Autodesk Fusion 360 part; units mm, degrees
(part 8 of 9)
  line L168 (107.3, 3.525) -> (107.3, 15.525)
  arc A160 (179.7375, 54.625) -> (178.7375, 53.625) centre (179.7375, 53.625) ccw
  line L169 (179.7375, 54.625) -> (191.7375, 54.625)
  arc A161 (192.7375, 53.625) -> (191.7375, 54.625) centre (191.7375, 53.625) ccw
  line L170 (192.7375, 53.625) -> (192.7375, 41.625)
  arc A162 (191.7375, 40.625) -> (192.7375, 41.625) centre (191.7375, 41.625) ccw
  line L171 (191.7375, 40.625) -> (179.7375, 40.625)
  arc A163 (178.7375, 41.625) -> (179.7375, 40.625) centre (179.7375, 41.625) ccw
  line L172 (178.7375, 41.625) -> (178.7375, 53.625)
  arc A164 (217.8375, 54.625) -> (216.8375, 53.625) centre (217.8375, 53.625) ccw
  line L173 (217.8375, 54.625) -> (229.8375, 54.625)
  arc A165 (230.8375, 53.625) -> (229.8375, 54.625) centre (229.8375, 53.625) ccw
  line L174 (230.8375, 53.625) -> (230.8375, 41.625)
  arc A166 (229.8375, 40.625) -> (230.8375, 41.625) centre (229.8375, 41.625) ccw
  line L175 (229.8375, 40.625) -> (217.8375, 40.625)
  arc A167 (216.8375, 41.625) -> (217.8375, 40.625) centre (217.8375, 41.625) ccw
  line L176 (216.8375, 41.625) -> (216.8375, 53.625)
  line L177 (229.1688, 22.575) -> (229.1688, 36.575)
  arc A168 (230.1688, 37.575) -> (229.1688, 36.575) centre (230.1688, 36.575) ccw
  line L178 (230.1688, 37.575) -> (236.1688, 37.575)
  arc A169 (237.1688, 36.575) -> (236.1688, 37.575) centre (236.1687, 36.575) ccw
  line L179 (237.1688, 36.575) -> (237.1688, 35.575)
  line L180 (237.1688, 35.575) -> (242.7688, 35.575)
  arc A170 (243.7688, 36.575) -> (242.7688, 35.575) centre (243.7688, 35.575) ccw
  line L181 (243.7688, 36.575) -> (246.7688, 36.575)
  arc A171 (247.7688, 35.575) -> (246.7688, 36.575) centre (246.7688, 35.575) ccw
  line L182 (247.7688, 35.575) -> (253.3688, 35.575)
  line L183 (253.3688, 35.575) -> (253.3688, 36.575)
  arc A172 (254.3688, 37.575) -> (253.3688, 36.575) centre (254.3688, 36.575) ccw
  line L184 (254.3688, 37.575) -> (260.3688, 37.575)
  arc A173 (261.3688, 36.575) -> (260.3688, 37.575) centre (260.3688, 36.575) ccw
  line L185 (261.3688, 36.575) -> (261.3688, 22.575)
  arc A174 (261.3687, 22.5664) -> (261.3688, 22.575) centre (260.3688, 22.575) ccw
  line L186 (261.3687, 22.5664) -> (261.3688, 22.5664)
  arc A175 (262.3688, 21.5664) -> (261.3688, 22.5664) centre (261.3688, 21.5664) ccw
  line L187 (262.3688, 21.5664) -> (262.3688, 16.525)
  line L188 (262.3688, 16.525) -> (263.175, 16.525)
  arc A176 (264.175, 15.525) -> (263.175, 16.525) centre (263.175, 15.525) ccw
  line L189 (264.175, 15.525) -> (264.175, 3.525)
  arc A177 (263.175, 2.525) -> (264.175, 3.525) centre (263.175, 3.525) ccw
  line L190 (263.175, 2.525) -> (251.175, 2.525)
  arc A178 (250.175, 3.525) -> (251.175, 2.525) centre (251.175, 3.525) ccw
  line L191 (250.175, 3.525) -> (250.175, 15.525)
  arc A179 (250.175, 15.525) -> (249.175, 16.525) centre (249.175, 15.525) ccw
  line L192 (249.175, 16.525) -> (241.3625, 16.525)
  arc A180 (241.3625, 16.525) -> (240.3625, 15.525) centre (241.3625, 15.525) ccw
  line L193 (240.3625, 15.525) -> (240.3625, 3.525)
  arc A181 (239.3625, 2.525) -> (240.3625, 3.525) centre (239.3625, 3.525) ccw
  line L194 (239.3625, 2.525) -> (227.3625, 2.525)
  arc A182 (226.3625, 3.525) -> (227.3625, 2.525) centre (227.3625, 3.525) ccw
  line L195 (226.3625, 3.525) -> (226.3625, 15.525)
  arc A183 (227.3625, 16.525) -> (226.3625, 15.525) centre (227.3625, 15.525) ccw
  line L196 (227.3625, 16.525) -> (228.1688, 16.525)
  line L197 (228.1688, 16.525) -> (228.1688, 21.5664)
  arc A184 (229.1688, 22.5664) -> (228.1688, 21.5664) centre (229.1688, 21.5664) ccw
  line L198 (229.1688, 22.5664) -> (229.1688, 22.5664)
  arc A185 (229.1688, 22.575) -> (229.1688, 22.5664) centre (230.1688, 22.575) ccw
  arc A186 (132.1125, 35.575) -> (131.1125, 34.575) centre (132.1125, 34.575) ccw
  line L199 (132.1125, 35.575) -> (144.1125, 35.575)
  arc A187 (145.1125, 34.575) -> (144.1125, 35.575) centre (144.1125, 34.575) ccw
  line L200 (145.1125, 34.575) -> (145.1125, 22.575)
  arc A188 (144.1125, 21.575) -> (145.1125, 22.575) centre (144.1125, 22.575) ccw
  line L201 (144.1125, 21.575) -> (132.1125, 21.575)
  arc A189 (131.1125, 22.575) -> (132.1125, 21.575) centre (132.1125, 22.575) ccw
  line L202 (131.1125, 22.575) -> (131.1125, 34.575)
  arc A190 (94.0125, 35.575) -> (93.0125, 34.575) centre (94.0125, 34.575) ccw
  line L203 (94.0125, 35.575) -> (106.0125, 35.575)
  arc A191 (107.0125, 34.575) -> (106.0125, 35.575) centre (106.0125, 34.575) ccw
  line L204 (107.0125, 34.575) -> (107.0125, 22.575)
  arc A192 (106.0125, 21.575) -> (107.0125, 22.575) centre (106.0125, 22.575) ccw
  line L205 (106.0125, 21.575) -> (94.0125, 21.575)
  arc A193 (93.0125, 22.575) -> (94.0125, 21.575) centre (94.0125, 22.575) ccw
  line L206 (93.0125, 22.575) -> (93.0125, 34.575)
  circle A194 centre (128.588, 37.025) radius 2
  circle A195 centre (220.025, 66.675) radius 2
  circle A196 centre (47.625, 9.525) radius 2
  circle A197 centre (245.269, 9.525) radius 2
  circle A198 centre (32.525, 66.675) radius 2
  line L207 (18.9313, 59.675) -> (23.9313, 59.675)
  line L208 (23.9313, 59.675) -> (23.9313, 58.675)
  line L209 (23.9313, 58.675) -> (18.9313, 58.675)
  line L210 (18.9313, 58.675) -> (18.9313, 59.675)
  line L211 (18.9313, 73.675) -> (23.9313, 73.675)
  line L212 (23.9313, 73.675) -> (23.9313, 74.675)
  line L213 (23.9313, 74.675) -> (18.9313, 74.675)
  line L214 (18.9313, 74.675) -> (18.9313, 73.675)
  line L215 (45.125, 59.675) -> (50.125, 59.675)
  line L216 (50.125, 59.675) -> (50.125, 58.675)
  line L217 (50.125, 58.675) -> (45.125, 58.675)
  line L218 (45.125, 58.675) -> (45.125, 59.675)
  line L219 (45.125, 73.675) -> (50.125, 73.675)
  line L220 (50.125, 73.675) -> (50.125, 74.675)
  line L221 (50.125, 74.675) -> (45.125, 74.675)
  line L222 (45.125, 74.675) -> (45.125, 73.675)
  line L223 (71.3188, 73.675) -> (76.3188, 73.675)
  line L224 (76.3188, 73.675) -> (76.3188, 74.675)
  line L225 (76.3188, 74.675) -> (71.3188, 74.675)
  line L226 (71.3188, 74.675) -> (71.3188, 73.675)
  line L227 (71.3188, 59.675) -> (76.3188, 59.675)
  line L228 (76.3188, 59.675) -> (76.3188, 58.675)
  line L229 (76.3188, 58.675) -> (71.3188, 58.675)
  line L230 (71.3188, 58.675) -> (71.3188, 59.675)
  line L231 (176.0937, 73.675) -> (181.0937, 73.675)
  line L232 (181.0937, 73.675) -> (181.0937, 74.675)
  line L233 (181.0937, 74.675) -> (176.0937, 74.675)
  line L234 (176.0937, 74.675) -> (176.0937, 73.675)
  line L235 (176.0938, 59.675) -> (181.0938, 59.675)
  line L236 (181.0938, 59.675) -> (181.0938, 58.675)
  line L237 (181.0938, 58.675) -> (176.0938, 58.675)
  line L238 (176.0938, 58.675) -> (176.0938, 59.675)
  line L239 (202.2875, 59.675) -> (207.2875, 59.675)
  line L240 (207.2875, 59.675) -> (207.2875, 58.675)
  line L241 (207.2875, 58.675) -> (202.2875, 58.675)
  line L242 (202.2875, 58.675) -> (202.2875, 59.675)
  line L243 (202.2875, 73.675) -> (207.2875, 73.675)
  line L244 (207.2875, 73.675) -> (207.2875, 74.675)
  line L245 (207.2875, 74.675) -> (202.2875, 74.675)
  line L246 (202.2875, 74.675) -> (202.2875, 73.675)
  line L247 (228.4813, 73.675) -> (233.4813, 73.675)
  line L248 (233.4813, 73.675) -> (233.4813, 74.675)
  line L249 (233.4813, 74.675) -> (228.4813, 74.675)
  line L250 (228.4813, 74.675) -> (228.4813, 73.675)
  line L251 (228.4812, 59.675) -> (233.4812, 59.675)
  line L252 (233.4812, 59.675) -> (233.4812, 58.675)
  line L253 (233.4812, 58.675) -> (228.4812, 58.675)
  line L254 (228.4812, 58.675) -> (228.4812, 59.675)
  line L255 (247.5312, 54.625) -> (252.5312, 54.625)
  line L256 (252.5312, 54.625) -> (252.5312, 55.625)
  line L257 (252.5312, 55.625) -> (247.5312, 55.625)
  line L258 (247.5312, 55.625) -> (247.5312, 54.625)
  line L259 (252.5312, 40.625) -> (247.5312, 40.625)
  line L260 (247.5312, 40.625) -> (247.5312, 39.625)
  line L261 (247.5312, 39.625) -> (252.5312, 39.625)
  line L262 (252.5312, 39.625) -> (252.5312, 40.625)
  line L263 (221.3375, 40.625) -> (226.3375, 40.625)
  line L264 (226.3375, 40.625) -> (226.3375, 39.625)
  line L265 (226.3375, 39.625) -> (221.3375, 39.625)
  line L266 (221.3375, 39.625) -> (221.3375, 40.625)
  line L267 (221.3375, 54.625) -> (226.3375, 54.625)
  line L268 (226.3375, 54.625) -> (226.3375, 55.625)
  line L269 (226.3375, 55.625) -> (221.3375, 55.625)
  line L270 (221.3375, 55.625) -> (221.3375, 54.625)
  line L271 (202.2875, 54.625) -> (207.2875, 54.625)
  line L272 (207.2875, 54.625) -> (207.2875, 55.625)
  line L273 (207.2875, 55.625) -> (202.2875, 55.625)
  line L274 (202.2875, 55.625) -> (202.2875, 54.625)
  line L275 (202.2875, 40.625) -> (207.2875, 40.625)
  line L276 (207.2875, 40.625) -> (207.2875, 39.625)
  line L277 (207.2875, 39.625) -> (202.2875, 39.625)
  line L278 (202.2875, 39.625) -> (202.2875, 40.625)
  line L279 (183.2375, 54.625) -> (188.2375, 54.625)
  line L280 (188.2375, 54.625) -> (188.2375, 55.625)
  line L281 (188.2375, 55.625) -> (183.2375, 55.625)
  line L282 (183.2375, 55.625) -> (183.2375, 54.625)
  line L283 (183.2375, 40.625) -> (188.2375, 40.625)
  line L284 (188.2375, 40.625) -> (188.2375, 39.625)
  line L285 (188.2375, 39.625) -> (183.2375, 39.625)
  line L286 (183.2375, 39.625) -> (183.2375, 40.625)
  line L287 (164.1875, 40.625) -> (169.1875, 40.625)
  line L288 (169.1875, 40.625) -> (169.1875, 39.625)
  line L289 (169.1875, 39.625) -> (164.1875, 39.625)
  line L290 (164.1875, 39.625) -> (164.1875, 40.625)
  line L291 (254.675, 2.525) -> (259.675, 2.525)
  line L292 (259.675, 2.525) -> (259.675, 1.525)
  line L293 (259.675, 1.525) -> (254.675, 1.525)
  line L294 (254.675, 1.525) -> (254.675, 2.525)
  line L295 (230.8625, 2.525) -> (235.8625, 2.525)
  line L296 (235.8625, 2.525) -> (235.8625, 1.525)
  line L297 (235.8625, 1.525) -> (230.8625, 1.525)
  line L298 (230.8625, 1.525) -> (230.8625, 2.525)
  line L299 (207.05, 2.525) -> (212.05, 2.525)
  line L300 (212.05, 2.525) -> (212.05, 1.525)
  line L301 (212.05, 1.525) -> (207.05, 1.525)
  line L302 (207.05, 1.525) -> (207.05, 2.525)
  line L303 (207.05, 16.525) -> (212.05, 16.525)
  line L304 (212.05, 16.525) -> (212.05, 17.525)
  line L305 (212.05, 17.525) -> (207.05, 17.525)
  line L306 (207.05, 17.525) -> (207.05, 16.525)
  line L307 (211.8125, 35.575) -> (216.8125, 35.575)
  line L308 (216.8125, 35.575) -> (216.8125, 36.575)
  line L309 (216.8125, 36.575) -> (211.8125, 36.575)
  line L310 (211.8125, 36.575) -> (211.8125, 35.575)
  line L311 (211.8125, 21.575) -> (216.8125, 21.575)
  line L312 (216.8125, 21.575) -> (216.8125, 20.575)
  line L313 (216.8125, 20.575) -> (211.8125, 20.575)
  line L314 (211.8125, 20.575) -> (211.8125, 21.575)
  line L315 (192.7625, 35.575) -> (197.7625, 35.575)
  line L316 (197.7625, 35.575) -> (197.7625, 36.575)
  line L317 (197.7625, 36.575) -> (192.7625, 36.575)
  line L318 (192.7625, 36.575) -> (192.7625, 35.575)
  line L319 (192.7625, 21.575) -> (197.7625, 21.575)
  line L320 (197.7625, 21.575) -> (197.7625, 20.575)
  line L321 (197.7625, 20.575) -> (192.7625, 20.575)
  line L322 (192.7625, 20.575) -> (192.7625, 21.575)
  line L323 (188, 16.525) -> (193, 16.525)
  line L324 (193, 16.525) -> (193, 17.525)
  line L325 (193, 17.525) -> (188, 17.525)
  line L326 (188, 17.525) -> (188, 16.525)
  line L327 (188, 2.525) -> (193, 2.525)
  line L328 (193, 2.525) -> (193, 1.525)
  line L329 (193, 1.525) -> (188, 1.525)
  line L330 (188, 1.525) -> (188, 2.525)
  line L331 (173.7125, 35.575) -> (178.7125, 35.575)
  line L332 (178.7125, 35.575) -> (178.7125, 36.575)
  line L333 (178.7125, 36.575) -> (173.7125, 36.575)
  line L334 (173.7125, 36.575) -> (173.7125, 35.575)
  line L335 (173.7125, 21.575) -> (178.7125, 21.575)
  line L336 (178.7125, 21.575) -> (178.7125, 20.575)
  line L337 (178.7125, 20.575) -> (173.7125, 20.575)
  line L338 (173.7125, 20.575) -> (173.7125, 21.575)
  line L339 (168.95, 16.525) -> (173.95, 16.525)
  line L340 (173.95, 16.525) -> (173.95, 17.525)
  line L341 (173.95, 17.525) -> (168.95, 17.525)
  line L342 (168.95, 17.525) -> (168.95, 16.525)
  line L343 (168.95, 2.525) -> (173.95, 2.525)
  line L344 (173.95, 2.525) -> (173.95, 1.525)
  line L345 (173.95, 1.525) -> (168.95, 1.525)
  line L346 (168.95, 1.525) -> (168.95, 2.525)
  line L347 (149.9, 16.525) -> (154.9, 16.525)
  line L348 (154.9, 16.525) -> (154.9, 17.525)
  line L349 (154.9, 17.525) -> (149.9, 17.525)
  line L350 (149.9, 17.525) -> (149.9, 16.525)
  line L351 (149.9, 2.525) -> (154.9, 2.525)
  line L352 (154.9, 2.525) -> (154.9, 1.525)
  line L353 (154.9, 1.525) -> (149.9, 1.525)
  line L354 (149.9, 1.525) -> (149.9, 2.525)
  line L355 (154.6625, 35.575) -> (159.6625, 35.575)
  line L356 (159.6625, 35.575) -> (159.6625, 36.575)
  line L357 (159.6625, 36.575) -> (154.6625, 36.575)
  line L358 (154.6625, 36.575) -> (154.6625, 35.575)
  line L359 (154.6625, 21.575) -> (159.6625, 21.575)
  line L360 (159.6625, 21.575) -> (159.6625, 20.575)
  line L361 (159.6625, 20.575) -> (154.6625, 20.575)
  line L362 (154.6625, 20.575) -> (154.6625, 21.575)
  line L363 (145.1375, 40.625) -> (150.1375, 40.625)
  line L364 (150.1375, 40.625) -> (150.1375, 39.625)
  line L365 (150.1375, 39.625) -> (145.1375, 39.625)
  line L366 (145.1375, 39.625) -> (145.1375, 40.625)
  line L367 (135.6125, 35.575) -> (140.6125, 35.575)
  line L368 (140.6125, 35.575) -> (140.6125, 36.575)
  line L369 (140.6125, 36.575) -> (135.6125, 36.575)
  line L370 (135.6125, 36.575) -> (135.6125, 35.575)
  line L371 (126.0875, 40.625) -> (131.0875, 40.625)
  line L372 (131.0875, 40.625) -> (131.0875, 39.625)
  line L373 (131.0875, 39.625) -> (126.0875, 39.625)
  line L374 (126.0875, 39.625) -> (126.0875, 40.625)
  line L375 (135.6125, 21.575) -> (140.6125, 21.575)
  line L376 (140.6125, 21.575) -> (140.6125, 20.575)
  line L377 (140.6125, 20.575) -> (135.6125, 20.575)
  line L378 (135.6125, 20.575) -> (135.6125, 21.575)
  line L379 (130.85, 16.525) -> (135.85, 16.525)
  line L380 (135.85, 16.525) -> (135.85, 17.525)
  line L381 (135.85, 17.525) -> (130.85, 17.525)
  line L382 (130.85, 17.525) -> (130.85, 16.525)
  line L383 (130.85, 2.525) -> (135.85, 2.525)
  line L384 (135.85, 2.525) -> (135.85, 1.525)
  line L385 (135.85, 1.525) -> (130.85, 1.525)
  line L386 (130.85, 1.525) -> (130.85, 2.525)
  line L387 (107.0375, 40.625) -> (112.0375, 40.625)
  line L388 (112.0375, 40.625) -> (112.0375, 39.625)
  line L389 (112.0375, 39.625) -> (107.0375, 39.625)
  line L390 (107.0375, 39.625) -> (107.0375, 40.625)
  line L391 (87.9875, 40.625) -> (92.9875, 40.625)
  line L392 (92.9875, 40.625) -> (92.9875, 39.625)
  line L393 (92.9875, 39.625) -> (87.9875, 39.625)
  line L394 (87.9875, 39.625) -> (87.9875, 40.625)
  line L395 (97.5125, 35.575) -> (102.5125, 35.575)
  line L396 (102.5125, 35.575) -> (102.5125, 36.575)
  line L397 (102.5125, 36.575) -> (97.5125, 36.575)
  line L398 (97.5125, 36.575) -> (97.5125, 35.575)
  line L399 (116.5625, 35.575) -> (121.5625, 35.575)
  line L400 (121.5625, 35.575) -> (121.5625, 36.575)
  line L401 (121.5625, 36.575) -> (116.5625, 36.575)
  line L402 (116.5625, 36.575) -> (116.5625, 35.575)
  line L403 (116.5625, 21.575) -> (121.5625, 21.575)
  line L404 (121.5625, 21.575) -> (121.5625, 20.575)
  line L405 (121.5625, 20.575) -> (116.5625, 20.575)
  line L406 (116.5625, 20.575) -> (116.5625, 21.575)
  line L407 (97.5125, 21.575) -> (102.5125, 21.575)
  line L408 (102.5125, 21.575) -> (102.5125, 20.575)
  line L409 (102.5125, 20.575) -> (97.5125, 20.575)
  line L410 (97.5125, 20.575) -> (97.5125, 21.575)
  line L411 (92.75, 16.525) -> (97.75, 16.525)
  line L412 (97.75, 16.525) -> (97.75, 17.525)
  line L413 (97.75, 17.525) -> (92.75, 17.525)
  line L414 (92.75, 17.525) -> (92.75, 16.525)
  line L415 (92.75, 2.525) -> (97.75, 2.525)
  line L416 (97.75, 2.525) -> (97.75, 1.525)
  line L417 (97.75, 1.525) -> (92.75, 1.525)
  line L418 (92.75, 1.525) -> (92.75, 2.525)
  line L419 (111.8, 16.525) -> (116.8, 16.525)
  line L420 (116.8, 16.525) -> (116.8, 17.525)
  line L421 (116.8, 17.525) -> (111.8, 17.525)
  line L422 (111.8, 17.525) -> (111.8, 16.525)
  line L423 (111.8, 2.525) -> (116.8, 2.525)
  line L424 (116.8, 2.525) -> (116.8, 1.525)
  line L425 (116.8, 1.525) -> (111.8, 1.525)
  line L426 (111.8, 1.525) -> (111.8, 2.525)
  line L427 (68.9375, 54.625) -> (73.9375, 54.625)
  line L428 (73.9375, 54.625) -> (73.9375, 55.625)
  line L429 (73.9375, 55.625) -> (68.9375, 55.625)
  line L430 (68.9375, 55.625) -> (68.9375, 54.625)
  line L431 (49.8875, 54.625) -> (54.8875, 54.625)
  line L432 (54.8875, 54.625) -> (54.8875, 55.625)
  line L433 (54.8875, 55.625) -> (49.8875, 55.625)
  line L434 (49.8875, 55.625) -> (49.8875, 54.625)
  line L435 (49.8875, 40.625) -> (54.8875, 40.625)
  line L436 (54.8875, 40.625) -> (54.8875, 39.625)
  line L437 (54.8875, 39.625) -> (49.8875, 39.625)
  line L438 (49.8875, 39.625) -> (49.8875, 40.625)
  line L439 (68.9375, 40.625) -> (73.9375, 40.625)
  line L440 (73.9375, 40.625) -> (73.9375, 39.625)
  line L441 (73.9375, 39.625) -> (68.9375, 39.625)
  line L442 (68.9375, 39.625) -> (68.9375, 40.625)
  line L443 (14.1688, 21.575) -> (19.1688, 21.575)
  line L444 (19.1688, 21.575) -> (19.1688, 20.575)
  line L445 (19.1688, 20.575) -> (14.1688, 20.575)
  line L446 (14.1688, 20.575) -> (14.1688, 21.575)
  line L447 (40.3625, 21.575) -> (45.3625, 21.575)
  line L448 (45.3625, 21.575) -> (45.3625, 20.575)
  line L449 (45.3625, 20.575) -> (40.3625, 20.575)
  line L450 (40.3625, 20.575) -> (40.3625, 21.575)
  line L451 (59.4125, 35.575) -> (64.4125, 35.575)
  line L452 (64.4125, 35.575) -> (64.4125, 36.575)
  line L453 (64.4125, 36.575) -> (59.4125, 36.575)
  line L454 (59.4125, 36.575) -> (59.4125, 35.575)
  line L455 (59.4125, 21.575) -> (64.4125, 21.575)
  line L456 (64.4125, 21.575) -> (64.4125, 20.575)
  line L457 (64.4125, 20.575) -> (59.4125, 20.575)
  line L458 (59.4125, 20.575) -> (59.4125, 21.575)
  line L459 (78.4625, 21.575) -> (83.4625, 21.575)
  line L460 (83.4625, 21.575) -> (83.4625, 20.575)
  line L461 (83.4625, 20.575) -> (78.4625, 20.575)
  line L462 (78.4625, 20.575) -> (78.4625, 21.575)
  line L463 (78.4625, 35.575) -> (83.4625, 35.575)
  line L464 (83.4625, 35.575) -> (83.4625, 36.575)
  line L465 (83.4625, 36.575) -> (78.4625, 36.575)
  line L466 (78.4625, 36.575) -> (78.4625, 35.575)
  line L467 (11.7875, 2.525) -> (16.7875, 2.525)
  line L468 (16.7875, 2.525) -> (16.7875, 1.525)
  line L469 (16.7875, 1.525) -> (11.7875, 1.525)
  line L470 (11.7875, 1.525) -> (11.7875, 2.525)
  line L471 (11.7875, 16.525) -> (16.7875, 16.525)
  line L472 (16.7875, 16.525) -> (16.7875, 17.525)
  line L473 (16.7875, 17.525) -> (11.7875, 17.525)
  line L474 (11.7875, 17.525) -> (11.7875, 16.525)
  line L475 (35.6, 16.525) -> (40.6, 16.525)
  line L476 (40.6, 16.525) -> (40.6, 17.525)
  line L477 (40.6, 17.525) -> (35.6, 17.525)
  line L478 (35.6, 17.525) -> (35.6, 16.525)
  line L479 (35.6, 2.525) -> (40.6, 2.525)
  line L480 (40.6, 2.525) -> (40.6, 1.525)
  line L481 (40.6, 1.525) -> (35.6, 1.525)
  line L482 (35.6, 1.525) -> (35.6, 2.525)
  line L483 (54.65, 2.525) -> (59.65, 2.525)
  line L484 (59.65, 2.525) -> (59.65, 1.525)
  line L485 (59.65, 1.525) -> (54.65, 1.525)
  line L486 (54.65, 1.525) -> (54.65, 2.525)
  line L487 (73.7, 2.525) -> (78.7, 2.525)
  line L488 (78.7, 2.525) -> (78.7, 1.525)
  line L489 (78.7, 1.525) -> (73.7, 1.525)
  line L490 (73.7, 1.525) -> (73.7, 2.525)
  line L491 (73.7, 16.525) -> (78.7, 16.525)
  line L492 (78.7, 16.525) -> (78.7, 17.525)
  line L493 (78.7, 17.525) -> (73.7, 17.525)
  line L494 (73.7, 17.525) -> (73.7, 16.525)
  line L495 (54.65, 16.525) -> (59.65, 16.525)
  line L496 (59.65, 16.525) -> (59.65, 17.525)
  line L497 (59.65, 17.525) -> (54.65, 17.525)
  line L498 (54.65, 17.525) -> (54.65, 16.525)
  dimension "d208" = 5
  dimension "d209" = 1
  dimension "d210" = 5
  dimension "d211" = 4.5
  dimension "d212" = 4.5
  dimension "d213" = 5
  dimension "d214" = 1
  dimension "d215" = 5
  dimension "d216" = 4.5
  dimension "d217" = 4.5
  dimension "d218" = 5
  dimension "d219" = 5
  dimension "d220" = 1
  dimension "d221" = 4.5
  dimension "d222" = 4.5
  dimension "d223" = 5
  dimension "d224" = 5
  dimension "d225" = 1
  dimension "d226" = 5
  dimension "d227" = 1
  dimension "d228" = 5
  dimension "d229" = 5
  dimension "d230" = 5
  dimension "d231" = 1
  dimension "d232" = 4.5
  dimension "d233" = 4.5
  dimension "d234" = 4.5
  dimension "d235" = 4.5
  dimension "d236" = 4.5
  dimension "d237" = 4.5
  dimension "d238" = 5
  dimension "d239" = 5
  dimension "d240" = 1
  dimension "d241" = 5
  dimension "d242" = 1
  dimension "d243" = 5
  dimension "d244" = 1
  dimension "d245" = 4.5
  dimension "d246" = 4.5
  dimension "d247" = 4.5
  dimension "d248" = 4.5
  dimension "d249" = 5
  dimension "d250" = 1
  dimension "d251" = 5
  dimension "d252" = 1
  dimension "d253" = 5
  dimension "d254" = 1
  dimension "d255" = 5
  dimension "d256" = 1
  dimension "d257" = 5
  dimension "d258" = 1
  dimension "d259" = 4.5
  dimension "d260" = 4.5
  dimension "d261" = 4.5
  dimension "d262" = 4.5
  dimension "d263" = 4.5
  dimension "d264" = 5
  dimension "d265" = 5
  dimension "d266" = 4.5
  dimension "d267" = 4.5
  dimension "d268" = 5
  dimension "d269" = 5
  dimension "d270" = 1
  dimension "d271" = 5
  dimension "d272" = 1
  dimension "d273" = 5
  dimension "d274" = 1
  dimension "d275" = 5
  dimension "d276" = 1
  dimension "d277" = 5
  dimension "d278" = 1
  dimension "d279" = 5
  dimension "d280" = 1
  dimension "d281" = 5
  dimension "d282" = 4.5
  dimension "d283" = 4.5
  dimension "d284" = 4.5
  dimension "d285" = 4.5
  dimension "d286" = 4.5
  dimension "d287" = 4.5
  dimension "d288" = 4.5
  dimension "d289" = 4.5
  dimension "d290" = 5
  dimension "d291" = 1
  dimension "d292" = 5
  dimension "d293" = 1
  dimension "d294" = 5
  dimension "d295" = 1
  dimension "d296" = 5
  dimension "d297" = 5
  dimension "d298" = 1
  dimension "d299" = 5
  dimension "d300" = 5
  dimension "d301" = 1
  dimension "d302" = 5
  dimension "d303" = 1
  dimension "d304" = 4.5
  dimension "d305" = 4.5
  dimension "d306" = 4.5
  dimension "d307" = 4.5
  dimension "d308" = 4.5
  dimension "d309" = 4.5
  dimension "d310" = 4.5
  dimension "d311" = 4.5
  dimension "d312" = 5
  dimension "d313" = 1
  dimension "d314" = 5
  dimension "d315" = 1
  dimension "d316" = 5
  dimension "d317" = 1
  dimension "d318" = 5
  dimension "d319" = 1
  dimension "d320" = 5
  dimension "d321" = 1
  dimension "d322" = 5
  dimension "d323" = 4.5
  dimension "d324" = 4.5
  dimension "d325" = 4.5
  dimension "d326" = 4.5
  dimension "d327" = 4.5
  dimension "d328" = 4.5
  dimension "d329" = 5
  dimension "d330" = 1
  dimension "d331" = 5
  dimension "d332" = 1
  dimension "d333" = 5
  dimension "d334" = 1
  dimension "d335" = 5
  dimension "d336" = 1
  dimension "d337" = 5
  dimension "d338" = 1
  dimension "d339" = 5
  dimension "d340" = 1
  dimension "d341" = 5
  dimension "d342" = 1
  dimension "d343" = 5
  dimension "d344" = 5
  dimension "d345" = 1
  dimension "d346" = 5
  dimension "d347" = 4.5
  dimension "d348" = 4.5
  dimension "d349" = 4.5
  dimension "d350" = 4.5
  dimension "d351" = 4.5
  dimension "d352" = 4.5
  dimension "d353" = 4.5
  dimension "d354" = 4.5
  dimension "d355" = 4.5
  dimension "d356" = 4.5
  dimension "d357" = 5
  dimension "d358" = 1
  dimension "d359" = 5
  dimension "d360" = 1
  dimension "d361" = 5
  dimension "d362" = 1
  dimension "d363" = 5
  dimension "d364" = 1
  dimension "d365" = 4.5
  dimension "d366" = 4.5
  dimension "d367" = 4.5
  dimension "d368" = 4.5
  dimension "d369" = 5
  dimension "d370" = 1
  dimension "d371" = 5
  dimension "d372" = 1
  dimension "d373" = 5
  dimension "d374" = 1
  dimension "d375" = 5
  dimension "d376" = 1
  dimension "d377" = 5
  dimension "d378" = 1
  dimension "d379" = 5
  dimension "d380" = 1
  dimension "d381" = 4.5
  dimension "d382" = 4.5
  dimension "d383" = 4.5
  dimension "d384" = 4.5
  dimension "d385" = 4.5
  dimension "d386" = 4.5
  dimension "d387" = 5
  dimension "d388" = 5
  dimension "d389" = 1
  dimension "d390" = 5
  dimension "d391" = 1
  dimension "d392" = 5
  dimension "d393" = 5
  dimension "d394" = 5
  dimension "d395" = 5
  dimension "d396" = 1
  dimension "d397" = 5
  dimension "d398" = 1
  dimension "d399" = 4.5
  dimension "d400" = 4.5
  dimension "d401" = 4.5
  dimension "d402" = 4.5
  dimension "d403" = 4.5
  dimension "d404" = 4.5
  dimension "d405" = 4.5
  dimension "d406" = 4.5
  constraint horizontal L207
  constraint vertical L208
  constraint horizontal L209
  constraint vertical L210
  constraint coincident L72 L207.start
  constraint horizontal L211
  constraint vertical L212
  constraint horizontal L213
  constraint vertical L214
  constraint coincident L70 L211.start
  constraint horizontal L215
  constraint vertical L216
  constraint horizontal L217
  constraint vertical L218
  constraint coincident L115 L215.start
  constraint horizontal L219
  constraint vertical L220
  constraint horizontal L221
  constraint vertical L222
  constraint coincident L113 L219.start
  constraint horizontal L223
  constraint vertical L224
  constraint horizontal L225
  constraint vertical L226
  constraint coincident L77 L223.start
  constraint horizontal L227
  constraint vertical L228
  constraint horizontal L229
  constraint vertical L230
  constraint coincident L79 L227.start
  constraint horizontal L231
  constraint vertical L232
  constraint horizontal L233
  constraint vertical L234
  constraint coincident L101 L231.start
  constraint horizontal L235
  constraint vertical L236
  constraint horizontal L237
  constraint vertical L238
  constraint coincident L103 L235.start
  constraint horizontal L239
  constraint vertical L240
  constraint horizontal L241
  constraint vertical L242
  constraint coincident L63 L239.start
  constraint horizontal L243
  constraint vertical L244
  constraint horizontal L245
  constraint vertical L246
  constraint coincident L61 L243.start
  constraint horizontal L247
  constraint vertical L248
  constraint horizontal L249
  constraint vertical L250
  constraint coincident L137 L247.start
  constraint horizontal L251
  constraint vertical L252
  constraint horizontal L253
  constraint vertical L254
  constraint coincident L139 L251.start
  constraint horizontal L255
  constraint vertical L256
  constraint horizontal L257
  constraint vertical L258
  constraint coincident L65 L255.start
  constraint horizontal L259
  constraint vertical L260
  constraint horizontal L261
  constraint vertical L262
  constraint coincident L67 L259.start
  constraint horizontal L263
  constraint vertical L264
  constraint horizontal L265
  constraint vertical L266
  constraint coincident L175 L263.start
  constraint horizontal L267
  constraint vertical L268
  constraint horizontal L269
  constraint vertical L270
  constraint coincident L173 L267.start
  constraint horizontal L271
  constraint vertical L272
  constraint horizontal L273
  constraint vertical L274
  constraint coincident L133 L271.start
  constraint horizontal L275
  constraint vertical L276
  constraint horizontal L277
  constraint vertical L278
  constraint coincident L135 L275.start
  constraint horizontal L279
  constraint vertical L280
  constraint horizontal L281
  constraint vertical L282
  constraint coincident L169 L279.start
  constraint horizontal L283
  constraint vertical L284
  constraint horizontal L285
  constraint vertical L286
  constraint coincident L171 L283.start
  constraint horizontal L287
  constraint vertical L288
  constraint horizontal L289
  constraint vertical L290
  constraint coincident L19 L287.start
  constraint horizontal L291
  constraint vertical L292
  constraint horizontal L293
  constraint vertical L294
  constraint coincident L190 L291.start
  constraint horizontal L295
  constraint vertical L296
  constraint horizontal L297
  constraint vertical L298
  constraint coincident L194 L295.start
  constraint horizontal L299
  constraint vertical L300
  constraint horizontal L301
  constraint vertical L302
  constraint coincident L163 L299.start
  constraint horizontal L303
  constraint vertical L304
  constraint horizontal L305
  constraint vertical L306
  constraint coincident L161 L303.start
  constraint horizontal L307
  constraint vertical L308
  constraint horizontal L309
  constraint vertical L310
  constraint coincident L121 L307.start
  constraint horizontal L311
  constraint vertical L312
  constraint horizontal L313
  constraint vertical L314
  constraint coincident L123 L311.start
  constraint horizontal L315
  constraint vertical L316
  constraint horizontal L317
  constraint vertical L318
  constraint coincident L157 L315.start
  constraint horizontal L319
  constraint vertical L320
  constraint horizontal L321
  constraint vertical L322
  constraint coincident L159 L319.start
  constraint horizontal L323
  constraint vertical L324
  constraint horizontal L325
  constraint vertical L326
  constraint coincident L81 L323.start
  constraint horizontal L327
  constraint vertical L328
  constraint horizontal L329
  constraint vertical L330
  constraint coincident L83 L327.start
  constraint horizontal L331
  constraint vertical L332
  constraint horizontal L333
  constraint vertical L334
  constraint coincident L141 L331.start
  constraint horizontal L335
  constraint vertical L336
  constraint horizontal L337
  constraint vertical L338
  constraint coincident L143 L335.start
  constraint horizontal L339
  constraint vertical L340
  constraint horizontal L341
  constraint vertical L342
  constraint coincident L73 L339.start
  constraint horizontal L343
  constraint vertical L344
  constraint horizontal L345
  constraint vertical L346
  constraint coincident L75 L343.start
  constraint horizontal L347
  constraint vertical L348
  constraint horizontal L349
  constraint vertical L350
  constraint coincident L153 L347.start
  constraint horizontal L351
  constraint vertical L352
  constraint horizontal L353
  constraint vertical L354
  constraint coincident L155 L351.start
  constraint horizontal L355
  constraint vertical L356
  constraint horizontal L357
  constraint vertical L358
  constraint coincident L105 L355.start
  constraint horizontal L359
  constraint vertical L360
  constraint horizontal L361
  constraint vertical L362
  constraint coincident L107 L359.start
  constraint horizontal L363
  constraint vertical L364
  constraint horizontal L365
  constraint vertical L366
  constraint coincident L23 L363.start
  constraint horizontal L367
  constraint vertical L368
  constraint horizontal L369
  constraint vertical L370
  constraint coincident L199 L367.start
  constraint horizontal L371
  constraint vertical L372
  constraint horizontal L373
  constraint vertical L374
  constraint coincident L27 L371.start
  constraint horizontal L375
  constraint vertical L376
  constraint horizontal L377
  constraint vertical L378
  constraint coincident L201 L375.start
  constraint horizontal L379
  constraint vertical L380
  constraint horizontal L381
  constraint vertical L382
  constraint coincident L145 L379.start
  constraint horizontal L383
  constraint vertical L384
  constraint horizontal L385
  constraint vertical L386
  constraint coincident L147 L383.start
  constraint horizontal L387
  constraint vertical L388
  constraint horizontal L389
  constraint vertical L390
  constraint coincident L31 L387.start
  constraint horizontal L391
  constraint vertical L392
  constraint horizontal L393
  constraint vertical L394
  constraint coincident L35 L391.start
  constraint horizontal L395
  constraint vertical L396
  constraint horizontal L397
  constraint vertical L398
  constraint coincident L203 L395.start
  constraint horizontal L399
  constraint vertical L400
  constraint horizontal L401
  constraint vertical L402
  constraint coincident L149 L399.start
  constraint horizontal L403
  constraint vertical L404
  constraint horizontal L405
  constraint vertical L406
  constraint coincident L151 L403.start
  constraint horizontal L407
  constraint vertical L408
  constraint horizontal L409
  constraint vertical L410
  constraint coincident L205 L407.start
  constraint horizontal L411
  constraint vertical L412
  constraint horizontal L413
  constraint vertical L414
  constraint coincident L109 L411.start
  constraint horizontal L415
  constraint vertical L416
  constraint horizontal L417
  constraint vertical L418
  constraint coincident L111 L415.start
  constraint horizontal L419
  constraint vertical L420
  constraint horizontal L421
  constraint vertical L422
  constraint coincident L165 L419.start
  constraint horizontal L423
  constraint vertical L424
  constraint horizontal L425
  constraint vertical L426
  constraint coincident L167 L423.start
  constraint horizontal L427
  constraint vertical L428
  constraint horizontal L429
  constraint vertical L430
  constraint coincident L57 L427.start
  constraint horizontal L431
  constraint vertical L432
  constraint horizontal L433
  constraint vertical L434
  constraint coincident L93 L431.start
  constraint horizontal L435
  constraint vertical L436
  constraint horizontal L437
  constraint vertical L438
  constraint coincident L95 L435.start
  constraint horizontal L439
  constraint vertical L440
  constraint horizontal L441
  constraint vertical L442
  constraint coincident L59 L439.start
  constraint horizontal L443
  constraint vertical L444
  constraint horizontal L445
  constraint vertical L446
  constraint coincident L2 L443.start
  constraint horizontal L447
  constraint vertical L448
  constraint horizontal L449
  constraint vertical L450
  constraint coincident L55 L447.start
  constraint horizontal L451
  constraint vertical L452
  constraint horizontal L453
  constraint vertical L454
  constraint coincident L89 L451.start
  constraint horizontal L455
  constraint vertical L456
  constraint horizontal L457
  constraint vertical L458
  constraint coincident L91 L455.start
  constraint horizontal L459
  constraint vertical L460
  constraint horizontal L461
  constraint vertical L462
  constraint coincident L119 L459.start
  constraint horizontal L463
  constraint vertical L464
  constraint horizontal L465
  constraint vertical L466
  constraint coincident L117 L463.start
  constraint horizontal L467
  constraint vertical L468
  constraint horizontal L469
  constraint vertical L470
  constraint coincident L127 L467.start
  constraint horizontal L471
  constraint vertical L472
  constraint horizontal L473
  constraint vertical L474
  constraint coincident L125 L471.start
  constraint horizontal L475
  constraint vertical L476
  constraint horizontal L477
  constraint vertical L478
  constraint coincident L88 L475.start
  constraint horizontal L479
  constraint vertical L480
  constraint horizontal L481
  constraint vertical L482
  constraint coincident L86 L479.start
  constraint horizontal L483
  constraint vertical L484
  constraint horizontal L485
  constraint vertical L486
  constraint coincident L131 L483.start
  constraint horizontal L487
  constraint vertical L488
  constraint horizontal L489
  constraint vertical L490
  constraint coincident L99 L487.start
  constraint horizontal L491
  constraint vertical L492
  constraint horizontal L493
  constraint vertical L494
  constraint coincident L97 L491.start
  constraint horizontal L495
  constraint vertical L496
  constraint horizontal L497
  constraint vertical L498
  constraint coincident L129 L495.start
  measures "d208" distance of L207.start L207.end
  measures "d209" distance of L207.start L209.end
  measures "d210" distance of L211.start L211.end
  measures "d211" distance of L69 L214
  measures "d212" distance of L69 L210
  measures "d213" distance of L215.start L215.end
  measures "d214" distance of L215.start L217.end
  measures "d215" distance of L219.start L219.end
  measures "d216" distance of L116 L222
  measures "d217" distance of L116 L218
  measures "d218" distance of L223.start L223.end
  measures "d219" distance of L227.start L227.end
  measures "d220" distance of L227.start L229.end
  measures "d221" distance of L80 L230
  measures "d222" distance of L80 L226
  measures "d223" distance of L231.start L231.end
  measures "d224" distance of L235.start L235.end
  measures "d225" distance of L235.start L237.end
  measures "d226" distance of L239.start L239.end
  measures "d227" distance of L239.start L241.end
  measures "d228" distance of L243.start L243.end
  measures "d229" distance of L247.start L247.end
  measures "d230" distance of L251.start L251.end
  measures "d231" distance of L251.start L253.end
  measures "d232" distance of L140 L254
  measures "d233" distance of L140 L250
  measures "d234" distance of L62 L244
  measures "d235" distance of L62 L240
  measures "d236" distance of L102 L236
  measures "d237" distance of L102 L232
  measures "d238" distance of L255.start L255.end
  measures "d239" distance of L259.start L259.end
  measures "d240" distance of L259.start L261.end
  measures "d241" distance of L263.start L263.end
  measures "d242" distance of L263.start L265.end
  measures "d243" distance of L267.start L267.end
  measures "d244" distance of L267.start L269.end
  measures "d245" distance of L68 L258
  measures "d246" distance of L68 L260
  measures "d247" distance of L174 L268
  measures "d248" distance of L174 L264
  measures "d249" distance of L271.start L271.end
  measures "d250" distance of L271.start L273.end
  measures "d251" distance of L275.start L275.end
  measures "d252" distance of L275.start L277.end
  measures "d253" distance of L279.start L279.end
  measures "d254" distance of L279.start L281.end
  measures "d255" distance of L283.start L283.end
  measures "d256" distance of L283.start L285.end
  measures "d257" distance of L287.start L287.end
  measures "d258" distance of L287.start L289.end
  measures "d259" distance of L134 L272
  measures "d260" distance of L134 L276
  measures "d261" distance of L170 L280
  measures "d262" distance of L170 L284
  measures "d263" distance of L18 L288
  measures "d264" distance of L291.start L291.end
  measures "d265" distance of L295.start L295.end
  measures "d266" distance of L193 L296
  measures "d267" distance of L191 L294
  measures "d268" distance of L299.start L299.end
  measures "d269" distance of L303.start L303.end
  measures "d270" distance of L303.start L305.end
  measures "d271" distance of L307.start L307.end
  measures "d272" distance of L307.start L309.end
  measures "d273" distance of L311.start L311.end
  measures "d274" distance of L311.start L313.end
  measures "d275" distance of L315.start L315.end
  measures "d276" distance of L315.start L317.end
  measures "d277" distance of L319.start L319.end
  measures "d278" distance of L319.start L321.end
  measures "d279" distance of L323.start L323.end
  measures "d280" distance of L323.start L325.end
  measures "d281" distance of L327.start L327.end
  measures "d282" distance of L162 L300
  measures "d283" distance of L162 L304
  measures "d284" distance of L122 L312
  measures "d285" distance of L122 L308
  measures "d286" distance of L158 L316
  measures "d287" distance of L158 L320
  measures "d288" distance of L82 L324
  measures "d289" distance of L82 L328
  measures "d290" distance of L331.start L331.end
  measures "d291" distance of L331.start L333.end
  measures "d292" distance of L335.start L335.end
  measures "d293" distance of L335.start L337.end
  measures "d294" distance of L339.start L339.end
  measures "d295" distance of L339.start L341.end
  measures "d296" distance of L343.start L343.end
  measures "d297" distance of L347.start L347.end
  measures "d298" distance of L347.start L349.end
  measures "d299" distance of L351.start L351.end
  measures "d300" distance of L355.start L355.end
  measures "d301" distance of L355.start L357.end
  measures "d302" distance of L359.start L359.end
  measures "d303" distance of L359.start L361.end
  measures "d304" distance of L74 L344
  measures "d305" distance of L74 L340
  measures "d306" distance of L154 L348
  measures "d307" distance of L154 L352
  measures "d308" distance of L142 L336
  measures "d309" distance of L142 L332
  measures "d310" distance of L106 L356
  measures "d311" distance of L106 L360
  measures "d312" distance of L363.start L363.end
  measures "d313" distance of L363.start L365.end
  measures "d314" distance of L367.start L367.end
  measures "d315" distance of L367.start L369.end
  measures "d316" distance of L371.start L371.end
  measures "d317" distance of L371.start L373.end
  measures "d318" distance of L375.start L375.end
  measures "d319" distance of L375.start L377.end
  measures "d320" distance of L379.start L379.end
  measures "d321" distance of L379.start L381.end
  measures "d322" distance of L383.start L383.end
  measures "d323" distance of L146 L384
  measures "d324" distance of L146 L380
  measures "d325" distance of L200 L376
  measures "d326" distance of L202 L370
  measures "d327" distance of L24 L366
  measures "d328" distance of L28 L374
  measures "d329" distance of L387.start L387.end
  measures "d330" distance of L387.start L389.end
  measures "d331" distance of L391.start L391.end
  measures "d332" distance of L391.start L393.end
  measures "d333" distance of L395.start L395.end
  measures "d334" distance of L395.start L397.end
  measures "d335" distance of L399.start L399.end
  measures "d336" distance of L399.start L401.end
  measures "d337" distance of L403.start L403.end
  measures "d338" distance of L403.start L405.end
  measures "d339" distance of L407.start L407.end
  measures "d340" distance of L407.start L409.end
  measures "d341" distance of L411.start L411.end
  measures "d342" distance of L411.start L413.end
  measures "d343" distance of L415.start L415.end
  measures "d344" distance of L419.start L419.end
  measures "d345" distance of L419.start L421.end
  measures "d346" distance of L423.start L423.end
  measures "d347" distance of L166 L424
  measures "d348" distance of L166 L420
  measures "d349" distance of L150 L404
  measures "d350" distance of L150 L400
  measures "d351" distance of L204 L408
  measures "d352" distance of L204 L396
  measures "d353" distance of L110 L416
  measures "d354" distance of L110 L412
  measures "d355" distance of L30 L388
  measures "d356" distance of L34 L392
  measures "d357" distance of L427.start L427.end
  measures "d358" distance of L427.start L429.end
  measures "d359" distance of L431.start L431.end
  measures "d360" distance of L431.start L433.end
  measures "d361" distance of L435.start L435.end
  measures "d362" distance of L435.start L437.end
  measures "d363" distance of L439.start L439.end
  measures "d364" distance of L439.start L441.end
  measures "d365" distance of L58 L440
  measures "d366" distance of L58 L428
  measures "d367" distance of L94 L432
  measures "d368" distance of L94 L436
  measures "d369" distance of L443.start L443.end
  measures "d370" distance of L443.start L445.end
  measures "d371" distance of L447.start L447.end
  measures "d372" distance of L447.start L449.end
  measures "d373" distance of L451.start L451.end
  measures "d374" distance of L451.start L453.end
  measures "d375" distance of L455.start L455.end
  measures "d376" distance of L455.start L457.end
  measures "d377" distance of L459.start L459.end
  measures "d378" distance of L459.start L461.end
  measures "d379" distance of L463.start L463.end
  measures "d380" distance of L463.start L465.end
  measures "d381" distance of L118 L464
  measures "d382" distance of L118 L460
  measures "d383" distance of L90 L456
  measures "d384" distance of L90 L452
  measures "d385" distance of L54 L448
  measures "d386" distance of L1 L444
  measures "d387" distance of L467.start L467.end
  measures "d388" distance of L471.start L471.end
  measures "d389" distance of L471.start L473.end
  measures "d390" distance of L475.start L475.end
  measures "d391" distance of L475.start L477.end
  measures "d392" distance of L479.start L479.end
  measures "d393" distance of L483.start L483.end
  measures "d394" distance of L487.start L487.end
  measures "d395" distance of L491.start L491.end
  measures "d396" distance of L491.start L493.end
  measures "d397" distance of L495.start L495.end
  measures "d398" distance of L495.start L497.end
  measures "d399" distance of L98 L492
  measures "d400" distance of L98 L488
  measures "d401" distance of L130 L484
  measures "d402" distance of L130 L496
  measures "d403" distance of L85 L476
  measures "d404" distance of L85 L480
  measures "d405" distance of L126 L472
  measures "d406" distance of L126 L468
extrude "Extrude13" cut sketch "Sketch14" against normal blind 3 contours L55 L447 L448 L449 L450 | L2 L443 L444 L445 L446 | L9 L127 L467 L468 L469 L470 | L9 L86 L479 L480 L481 L482 | L9 L131 L483 L484 L485 L486 | L9 L99 L487 L488 L489 L490 | L125 L471 L472 L473 L474 | L9 L111 L415 L416 L417 L418 | L88 L475 L476 L477 L478 | L9 L167 L423 L424 L425 L426 | L129 L495 L496 L497 L498 | L41 L70 L211 L212 L213 L214 | L9 L147 L383 L384 L385 L386 | L97 L491 L492 L493 L494 | L41 L113 L219 L220 L221 L222 | L9 L155 L351 L352 L353 L354 | L109 L411 L412 L413 L414 | L41 L77 L223 L224 L225 L226 | L9 L75 L343 L344 L345 L346 | L165 L419 L420 L421 L422 | L72 L207 L208 L209 L210 | L9 L83 L327 L328 L329 L330 | L145 L379 L380 L381 L382 | L115 L215 L216 L217 L218 | L9 L163 L299 L300 L301 L302 | L153 L347 L348 L349 L350 | L79 L227 L228 L229 L230 | L9 L194 L295 L296 L297 L298 | L73 L339 L340 L341 L342 | L9 L190 L291 L292 L293 L294 | L81 L323 L324 L325 L326 | L161 L303 L304 L305 L306 | L35 L391 L392 L393 L394 | L11 L65 L255 L256 L257 L258 | L13 L137 L247 L248 L249 L250 | L67 L259 L260 L261 L262 | L31 L387 L388 L389 L390 | L13 L61 L243 L244 L245 L246 | L13 L101 L231 L232 L233 L234 | L139 L251 L252 L253 L254 | L63 L239 L240 L241 L242 | L103 L235 L236 L237 L238 | L27 L371 L372 L373 L374 | L19 L287 L288 L289 L290 | L23 L363 L364 L365 L366 | L57 L427 L428 L429 L430 | L59 L439 L440 L441 L442 | L89 L451 L452 L453 L454 | L91 L455 L456 L457 L458 | L93 L431 L432 L433 L434 | L95 L435 L436 L437 L438 | L105 L355 L356 L357 L358 | L107 L359 L360 L361 L362 | L117 L463 L464 L465 L466 | L119 L459 L460 L461 L462 | L121 L307 L308 L309 L310 | L123 L311 L312 L313 L314 | L133 L271 L272 L273 L274 | L135 L275 L276 L277 L278 | L141 L331 L332 L333 L334 | L143 L335 L336 L337 L338 | L149 L399 L400 L401 L402 | L151 L403 L404 L405 L406 | L157 L315 L316 L317 L318 | L159 L319 L320 L321 L322 | L169 L279 L280 L281 L282 | L171 L283 L284 L285 L286 | L173 L267 L268 L269 L270 | L175 L263 L264 L265 L266 | L199 L367 L368 L369 L370 | L201 L375 L376 L377 L378 | L203 L395 L396 L397 L398 | L205 L407 L408 L409 L410
fillet "Fillet11" radius 1 9 edges at (4.3312, 2.1, 35.575) (14.1688, 2.1, 20.575) (19.1688, 2.1, 20.575) (11.7875, 2.1, 1.525) (16.7875, 2.1, 1.525) (11.7875, 2.1, 17.525) (16.7875, 2.1, 17.525) (18.9313, 2.1, 58.675) (23.9313, 2.1, 58.675)
fillet "Fillet12" radius 1 2 edges at (18.9313, 2.1, 74.675) (23.9313, 2.1, 74.675)
fillet "Fillet13" radius 1 8 edges at (45.125, 2.1, 74.675) (50.125, 2.1, 74.675) (45.125, 2.1, 58.675) (50.125, 2.1, 58.675) (71.3188, 2.1, 58.675) (71.3188, 2.1, 74.675) (76.3188, 2.1, 74.675) (76.3188, 2.1, 58.675)
fillet "Fillet14" radius 1 12 edges at (181.0938, 2.1, 58.675) (176.0938, 2.1, 58.675) (176.0937, 2.1, 74.675) (181.0937, 2.1, 74.675) (202.2875, 2.1, 74.675) (207.2875, 2.1, 74.675) (207.2875, 2.1, 58.675) (202.2875, 2.1, 58.675) (228.4812, 2.1, 58.675) (233.4813, 2.1, 74.675) (228.4813, 2.1, 74.675) (233.4812, 2.1, 58.675)